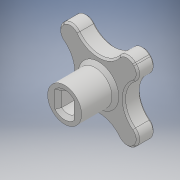
# Autodesk Inventor part: Reverse_knob_v1
Saved by Autodesk Inventor 2018 (Build 220112000, 112)
## iProperties
Created: 2018-02-15
Part Number: Reverse_knob_v1
Material: Generic
Document SubType Name: Modeling
Designer: jan-j
Density: 1 g/cm^3
Appearance: Default
Author: jan-j
Autodesk Inventor part; units mm, degrees
ref_plane "YZ Plane" through (0, 0, 0) normal (1, 0, 0) x (0, 1, 0)
ref_plane "XZ Plane" through (0, 0, 0) normal (0, 1, 0) x (-1, 0, 0)
ref_plane "XY Plane" through (0, 0, 0) normal (0, 0, 1) x (1, 0, 0)
sketch "Sketch1" plane through (0, 0, 0) normal (0, 1, 0) x (-1, 0, 0)
  spline S0 degree 3 poles (52.003, 82.0748) (54.2729, 82.1415) (56.1672, 80.3553) (56.2339, 78.0854) knots 0 0 0 0 0.2 0.2 0.2 0.2
  line L0 (52.003, 82.0748) -> (54.2729, 82.1415) construction
  line L1 (54.2729, 82.1415) -> (56.1672, 80.3553) construction
  line L2 (56.1672, 80.3553) -> (56.2339, 78.0854) construction
  spline S1 degree 3 poles (56.2339, 78.0854) (56.234, 78.0831) (56.3005, 75.8155) (54.5144, 73.9212) (52.2444, 73.8545) knots 0.2 0.2 0.2 0.2 0.2 0.4 0.4 0.4 0.4
  line L3 (56.2339, 78.0854) -> (56.2339, 78.0854) construction
  line L4 (56.2339, 78.0854) -> (56.3005, 75.8155) construction
  line L5 (56.3005, 75.8155) -> (54.5144, 73.9212) construction
  line L6 (54.5144, 73.9212) -> (52.2444, 73.8545) construction
  spline S2 degree 3 poles (52.2444, 73.8545) (52.2421, 73.8544) (49.9745, 73.7879) (48.0802, 75.574) (48.0136, 77.844) knots 0.4 0.4 0.4 0.4 0.4 0.6 0.6 0.6 0.6
  line L7 (52.2444, 73.8545) -> (52.2444, 73.8545) construction
  line L8 (52.2444, 73.8545) -> (49.9745, 73.7879) construction
  line L9 (49.9745, 73.7879) -> (48.0802, 75.574) construction
  line L10 (48.0802, 75.574) -> (48.0136, 77.844) construction
  spline S3 degree 3 poles (48.0136, 77.844) (48.0135, 77.8463) (47.9469, 80.1139) (49.7331, 82.0082) (52.003, 82.0748) knots 0.6 0.6 0.6 0.6 0.6 1 1 1 1
  line L11 (48.0136, 77.844) -> (48.0136, 77.844) construction
  line L12 (48.0136, 77.844) -> (47.9469, 80.1139) construction
  line L13 (47.9469, 80.1139) -> (49.7331, 82.0082) construction
  line L14 (49.7331, 82.0082) -> (52.003, 82.0748) construction
  spline S4 degree 3 poles (52.043, 80.7135) (52.7551, 80.7344) (53.4119, 80.4827) (53.9132, 80.0528) knots 0 0 0 0 0.142857 0.142857 0.142857 0.142857
  line L15 (52.043, 80.7135) -> (52.7551, 80.7344) construction
  line L16 (52.7551, 80.7344) -> (53.4119, 80.4827) construction
  line L17 (53.4119, 80.4827) -> (53.9132, 80.0528) construction
  line L18 (53.9132, 80.0528) -> (54.0327, 75.9851)
  spline S5 degree 3 poles (54.0327, 75.9851) (54.0322, 75.9846) (53.5575, 75.5266) (52.9166, 75.2368) (52.2045, 75.2158) knots 0.285714 0.285714 0.285714 0.285714 0.285714 0.428571 0.428571 0.428571 0.428571
  line L19 (54.0327, 75.9851) -> (54.0327, 75.9851) construction
  line L20 (54.0327, 75.9851) -> (53.5575, 75.5266) construction
  line L21 (53.5575, 75.5266) -> (52.9166, 75.2368) construction
  line L22 (52.9166, 75.2368) -> (52.2045, 75.2158) construction
  spline S6 degree 3 poles (52.2045, 75.2158) (52.2038, 75.2158) (51.4924, 75.1949) (50.8356, 75.4467) (50.3343, 75.8765) knots 0.428571 0.428571 0.428571 0.428571 0.428571 0.571429 0.571429 0.571429 0.571429
  line L23 (52.2045, 75.2158) -> (52.2045, 75.2158) construction
  line L24 (52.2045, 75.2158) -> (51.4924, 75.1949) construction
  line L25 (51.4924, 75.1949) -> (50.8356, 75.4467) construction
  line L26 (50.8356, 75.4467) -> (50.3343, 75.8765) construction
  line L27 (50.3343, 75.8765) -> (50.2148, 79.9442)
  spline S7 degree 3 poles (50.2148, 79.9442) (50.2153, 79.9447) (50.6901, 80.4027) (51.331, 80.6926) (52.043, 80.7135) knots 0.714286 0.714286 0.714286 0.714286 0.714286 1 1 1 1
  line L28 (50.2148, 79.9442) -> (50.2148, 79.9442) construction
  line L29 (50.2148, 79.9442) -> (50.6901, 80.4027) construction
  line L30 (50.6901, 80.4027) -> (51.331, 80.6926) construction
  line L31 (51.331, 80.6926) -> (52.043, 80.7135) construction
  line L32 (51.2109, 84.7632) -> (50.7914, 84.7226)
  line L33 (50.7914, 84.7226) -> (50.3879, 84.6009)
  line L34 (50.3879, 84.6009) -> (50.2754, 84.408)
  line L35 (50.2754, 84.408) -> (50.0351, 83.5249)
  line L36 (50.0351, 83.5249) -> (50.0328, 82.9691)
  line L37 (50.0328, 82.9691) -> (50.0829, 82.7792)
  line L38 (50.0829, 82.7792) -> (50.4014, 82.2224)
  line L39 (50.4014, 82.2224) -> (50.3612, 81.7237)
  line L40 (50.3612, 81.7237) -> (49.3357, 81.041)
  line L41 (49.3357, 81.041) -> (48.8601, 81.1964)
  line L42 (48.8601, 81.1964) -> (48.4694, 81.705)
  line L43 (48.4694, 81.705) -> (48.3135, 81.8245)
  line L44 (48.3135, 81.8245) -> (47.7998, 82.0368)
  line L45 (47.7998, 82.0368) -> (46.8924, 82.1558)
  line L46 (46.8924, 82.1558) -> (46.671, 82.1265)
  line L47 (46.671, 82.1265) -> (46.403, 81.8012)
  line L48 (46.403, 81.8012) -> (46.2038, 81.4298)
  line L49 (46.2038, 81.4298) -> (46.2607, 81.2139)
  line L50 (46.2607, 81.2139) -> (46.7151, 80.4194)
  line L51 (46.7151, 80.4194) -> (47.1065, 80.0248)
  line L52 (47.1065, 80.0248) -> (47.2763, 79.926)
  line L53 (47.2763, 79.926) -> (47.8952, 79.7575)
  line L54 (47.8952, 79.7575) -> (48.2194, 79.3764)
  line L55 (48.2194, 79.3764) -> (47.977, 78.1686)
  line L56 (47.977, 78.1686) -> (47.5309, 77.9421)
  line L57 (47.5309, 77.9421) -> (46.8948, 78.0255)
  line L58 (46.8948, 78.0255) -> (46.7002, 77.9997)
  line L59 (46.7002, 77.9997) -> (46.1868, 77.7868)
  line L60 (46.1868, 77.7868) -> (45.4611, 77.2291)
  line L61 (45.4611, 77.2291) -> (45.3252, 77.0518)
  line L62 (45.3252, 77.0518) -> (45.3658, 76.6324)
  line L63 (45.3658, 76.6324) -> (45.4874, 76.2289)
  line L64 (45.4874, 76.2289) -> (45.6804, 76.1164)
  line L65 (45.6804, 76.1164) -> (46.5635, 75.876)
  line L66 (46.5635, 75.876) -> (47.1193, 75.8738)
  line L67 (47.1193, 75.8738) -> (47.3092, 75.9239)
  line L68 (47.3092, 75.9239) -> (47.8659, 76.2424)
  line L69 (47.8659, 76.2424) -> (48.3647, 76.2021)
  line L70 (48.3647, 76.2021) -> (49.0474, 75.1767)
  line L71 (49.0474, 75.1767) -> (48.892, 74.7011)
  line L72 (48.892, 74.7011) -> (48.3834, 74.3103)
  line L73 (48.3834, 74.3103) -> (48.2639, 74.1545)
  line L74 (48.2639, 74.1545) -> (48.0515, 73.6408)
  line L75 (48.0515, 73.6408) -> (47.9326, 72.7334)
  line L76 (47.9326, 72.7334) -> (47.9619, 72.5119)
  line L77 (47.9619, 72.5119) -> (48.2872, 72.244)
  line L78 (48.2872, 72.244) -> (48.6585, 72.0447)
  line L79 (48.6585, 72.0447) -> (48.8745, 72.1016)
  line L80 (48.8745, 72.1016) -> (49.669, 72.5561)
  line L81 (49.669, 72.5561) -> (50.0635, 72.9475)
  line L82 (50.0635, 72.9475) -> (50.1624, 73.1172)
  line L83 (50.1624, 73.1172) -> (50.3309, 73.7361)
  line L84 (50.3309, 73.7361) -> (50.712, 74.0604)
  line L85 (50.712, 74.0604) -> (51.9197, 73.818)
  line L86 (51.9197, 73.818) -> (52.1463, 73.3718)
  line L87 (52.1463, 73.3718) -> (52.0629, 72.7358)
  line L88 (52.0629, 72.7358) -> (52.0886, 72.5411)
  line L89 (52.0886, 72.5411) -> (52.3016, 72.0277)
  line L90 (52.3016, 72.0277) -> (52.8592, 71.302)
  line L91 (52.8592, 71.302) -> (53.0365, 71.1661)
  line L92 (53.0365, 71.1661) -> (53.456, 71.2067)
  line L93 (53.456, 71.2067) -> (53.8595, 71.3284)
  line L94 (53.8595, 71.3284) -> (53.9719, 71.5214)
  line L95 (53.9719, 71.5214) -> (54.2124, 72.4044)
  line L96 (54.2124, 72.4044) -> (54.2146, 72.9603)
  line L97 (54.2146, 72.9603) -> (54.1645, 73.1502)
  line L98 (54.1645, 73.1502) -> (53.846, 73.7069)
  line L99 (53.846, 73.7069) -> (53.8862, 74.2056)
  line L100 (53.8862, 74.2056) -> (54.9117, 74.8883)
  line L101 (54.9117, 74.8883) -> (55.3873, 74.733)
  line L102 (55.3873, 74.733) -> (55.778, 74.2243)
  line L103 (55.778, 74.2243) -> (55.9339, 74.1049)
  line L104 (55.9339, 74.1049) -> (56.4476, 73.8925)
  line L105 (56.4476, 73.8925) -> (57.355, 73.7736)
  line L106 (57.355, 73.7736) -> (57.5765, 73.8028)
  line L107 (57.5765, 73.8028) -> (57.8444, 74.1282)
  line L108 (57.8444, 74.1282) -> (58.0436, 74.4995)
  line L109 (58.0436, 74.4995) -> (57.9867, 74.7155)
  line L110 (57.9867, 74.7155) -> (57.5323, 75.5099)
  line L111 (57.5323, 75.5099) -> (57.1408, 75.9045)
  line L112 (57.1408, 75.9045) -> (56.9711, 76.0033)
  line L113 (56.9711, 76.0033) -> (56.3523, 76.1718)
  line L114 (56.3523, 76.1718) -> (56.028, 76.553)
  line L115 (56.028, 76.553) -> (56.2704, 77.7607)
  line L116 (56.2704, 77.7607) -> (56.7165, 77.9872)
  line L117 (56.7165, 77.9872) -> (57.3526, 77.9039)
  line L118 (57.3526, 77.9039) -> (57.5472, 77.9296)
  line L119 (57.5472, 77.9296) -> (58.0606, 78.1426)
  line L120 (58.0606, 78.1426) -> (58.7864, 78.7002)
  line L121 (58.7864, 78.7002) -> (58.9223, 78.8775)
  line L122 (58.9223, 78.8775) -> (58.8816, 79.297)
  line L123 (58.8816, 79.297) -> (58.7599, 79.7005)
  line L124 (58.7599, 79.7005) -> (58.567, 79.8129)
  line L125 (58.567, 79.8129) -> (57.6839, 80.0533)
  line L126 (57.6839, 80.0533) -> (57.1281, 80.0556)
  line L127 (57.1281, 80.0556) -> (56.9382, 80.0055)
  line L128 (56.9382, 80.0055) -> (56.3815, 79.687)
  line L129 (56.3815, 79.687) -> (55.8827, 79.7272)
  line L130 (55.8827, 79.7272) -> (55.2, 80.7526)
  line L131 (55.2, 80.7526) -> (55.3554, 81.2283)
  line L132 (55.3554, 81.2283) -> (55.864, 81.619)
  line L133 (55.864, 81.619) -> (55.9835, 81.7749)
  line L134 (55.9835, 81.7749) -> (56.1959, 82.2886)
  line L135 (56.1959, 82.2886) -> (56.3148, 83.196)
  line L136 (56.3148, 83.196) -> (56.2855, 83.4174)
  line L137 (56.2855, 83.4174) -> (55.9602, 83.6853)
  line L138 (55.9602, 83.6853) -> (55.5889, 83.8846)
  line L139 (55.5889, 83.8846) -> (55.3729, 83.8277)
  line L140 (55.3729, 83.8277) -> (54.5784, 83.3733)
  line L141 (54.5784, 83.3733) -> (54.1839, 82.9818)
  line L142 (54.1839, 82.9818) -> (54.085, 82.8121)
  line L143 (54.085, 82.8121) -> (53.9165, 82.1932)
  line L144 (53.9165, 82.1932) -> (53.5354, 81.8689)
  line L145 (53.5354, 81.8689) -> (52.3277, 82.1114)
  line L146 (52.3277, 82.1114) -> (52.1012, 82.5575)
  line L147 (52.1012, 82.5575) -> (52.1845, 83.1935)
  line L148 (52.1845, 83.1935) -> (52.1588, 83.3882)
  line L149 (52.1588, 83.3882) -> (51.9458, 83.9016)
  line L150 (51.9458, 83.9016) -> (51.3881, 84.6273)
  line L151 (51.3881, 84.6273) -> (51.2109, 84.7632)
  circle A0 centre (0, 0) radius 2.85
  line L152 (0, 2.85) -> (0, -2.85)
  line L153 (-1.85, 2.1679) -> (-1.85, -2.1679)
  line L154 (1.85, -2.1679) -> (1.85, 2.1679)
  circle A1 centre (0, 0) radius 5
  dimension "d1" = 5.7
  dimension "d3" = 3.7
  dimension "d4" = 10
  constraints: 250 end point, 6 point on circle, 2 centre point, 2 coincident, 1 midpoint, 1 parallel, 1 vertical, 25 other
  measures "d1" diameter of A0
  measures "d3" distance between parallel lines of L153 L154
  measures "d4" diameter of A1
extrude "Extrusion1" add sketch "Sketch1" along normal blind 10 contours A0 L154 | L153 A0 | A1
sketch "Sketch2" plane through (0, 10, 0) normal (0, 1, 0) x (1, 0, 0)
  circle A0 centre (0, 0) radius 15
  dimension "d7" = 30
  constraints: 1 centre point, 1 coincident
  measures "d7" diameter of A0
extrude "Extrusion2" add sketch "Sketch2" along normal blind 5
sketch "Sketch3" plane through (0, 15, 0) normal (0, 1, 0) x (1, 0, 0)
  circle A0 centre (0, 0) radius 15 projected
  circle A1 centre (0, 15) radius 7.5
  line L0 (0, 15) -> (0, 0)
  dimension "d10" = 15
  constraints: 2 end point, 1 centre point, 1 vertical, 1 vertical alignment, 1 other
  measures "d10" diameter of A1
extrude "Extrusion3" cut sketch "Sketch3" against normal blind 5 contours A1 L0 A0 | A0 A1 | A0 L0 A1 picked at (1.7156, 17.2702)
fillet "Fillet1" radius 3 2 edges at (-7.2618, 12.5, -13.125) (7.2618, 12.5, -13.125)
pattern_circular "Circular Pattern1" count 4 over 360 about axis through (0, 0, 0) along (0, 1, 0) of "Extrusion3", "Fillet1"
chamfer "Chamfer1" distance 1 angle 45 4 edges at (-1.85, 0, 0) (0, 0, 2.85) (0, 0, -2.85) (1.85, 0, 0)
chamfer "Chamfer2" distance 1 angle 45 1 edges at (5, 10, 0)
chamfer "Chamfer3" distance 0.5 angle 45 32 edges at (-7.5, 10, 0) (-11.6166, 10, -8.1191) (-11.6166, 10, 8.1191) (-10.6066, 10, -10.6066) (8.1191, 10, -11.6166) (-8.1191, 10, -11.6166) (0, 10, -7.5) (10.6066, 10, -10.6066) (11.6166, 10, -8.1191) (11.6166, 10, 8.1191) (7.5, 10, 0) (10.6066, 10, 10.6066) (8.1191, 10, 11.6166) (-8.1191, 10, 11.6166) (0, 10, 7.5) (-10.6066, 10, 10.6066) (0, 15, 7.5) (8.1191, 15, 11.6166) (-8.1191, 15, 11.6166) (10.6066, 15, 10.6066) (11.6166, 15, -8.1191) (11.6166, 15, 8.1191) (7.5, 15, 0) (10.6066, 15, -10.6066) (8.1191, 15, -11.6166) (-8.1191, 15, -11.6166) (0, 15, -7.5) (-10.6066, 15, -10.6066) (-11.6166, 15, -8.1191) (-11.6166, 15, 8.1191) (-7.5, 15, 0) (-10.6066, 15, 10.6066)
body "Solid1"
